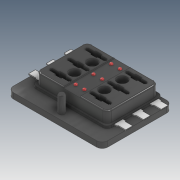
# Autodesk Inventor part: Fuse Box 6-way
Saved by Autodesk Inventor 2020 (Build 240168000, 168)
## iProperties
Created: 2021-05-27
Part Number: Fuse Box 6-way
Material: Generic
Document SubType Name: Modeling
Designer: Simon.Alvarez
Density: 1 g/cm^3
Appearance: Default
Author: Simon.Alvarez
Autodesk Inventor part; units mm, degrees
ref_plane "YZ Plane" through (0, 0, 0) normal (1, 0, 0) x (0, 1, 0)
ref_plane "XZ Plane" through (0, 0, 0) normal (0, 1, 0) x (-1, 0, 0)
ref_plane "XY Plane" through (0, 0, 0) normal (0, 0, 1) x (1, 0, 0)
sketch "Sketch1" plane through (0, 0, 0) normal (0, 1, 0) x (-1, 0, 0)
  line L0 (37.5, 31.5) -> (-37.5, 31.5)
  line L1 (-42.5, 26.5) -> (-42.5, -26.5)
  line L2 (-37.5, -31.5) -> (37.5, -31.5)
  line L3 (42.5, -26.5) -> (42.5, 26.5)
  line L4 (42.5, 31.5) -> (-42.5, -31.5) construction
  line L5 (-42.5, 31.5) -> (42.5, -31.5) construction
  arc A0 (42.5, 26.5) -> (37.5, 31.5) centre (37.5, 26.5) ccw
  arc A1 (-37.5, 31.5) -> (-42.5, 26.5) centre (-37.5, 26.5) ccw
  arc A2 (-42.5, -26.5) -> (-37.5, -31.5) centre (-37.5, -26.5) ccw
  arc A3 (37.5, -31.5) -> (42.5, -26.5) centre (37.5, -26.5) ccw
  point P0 (0, 0)
  dimension "d0" = 85
  dimension "d1" = 63
  dimension "d2" = 5
  constraints: 12 end point, 8 point on circle, 8 point on line, 8 tangent, 4 centre point, 3 equal radius, 2 midpoint, 2 parallel, 1 horizontal, 1 perpendicular
  measures "d0" distance of L4.end L5.end
  measures "d1" distance of L5.end L4.start
  measures "d2" radius of A0
extrude "Extrusion1" add sketch "Sketch1" along normal blind 5
sketch "Sketch2" plane through (0, 5, 0) normal (0, 1, 0) x (1, 0, 0)
  line L0 (37.5, 31.5) -> (-37.5, 31.5) projected
  line L1 (-30, 31.5) -> (30, 31.5)
  line L2 (34, 27.5) -> (34, -14.5)
  line L3 (30, -18.5) -> (-30, -18.5)
  line L4 (-34, -14.5) -> (-34, 27.5)
  line L5 (-42.5, 26.5) -> (-42.5, -26.5) projected
  line L6 (42.5, -26.5) -> (42.5, 26.5) projected
  line L7 (-37.5, -31.5) -> (37.5, -31.5) projected
  arc A0 (-34, -14.5) -> (-30, -18.5) centre (-30, -14.5) ccw
  arc A1 (30, -18.5) -> (34, -14.5) centre (30, -14.5) ccw
  arc A2 (34, 27.5) -> (30, 31.5) centre (30, 27.5) ccw
  arc A3 (-30, 31.5) -> (-34, 27.5) centre (-30, 27.5) ccw
  point P0 (0, 0)
  point P1 (-34, 31.5)
  point P2 (30, 31.5)
  dimension "d6" = 8.5
  dimension "d7" = 8.5
  dimension "d8" = 13
  dimension "d9" = 4
  constraints: 8 end point, 8 point on circle, 8 tangent, 4 centre point, 3 equal radius, 3 point on line, 2 parallel, 1 horizontal, 1 perpendicular
  measures "d6" distance between parallel lines of L5 L4
  measures "d7" distance between parallel lines of L6 L2
  measures "d8" distance between parallel lines of L7 L3
  measures "d9" radius of A0
extrude "Extrusion2" add sketch "Sketch2" along normal blind 2
sketch "Sketch3" plane through (0, 7, 0) normal (0, 1, 0) x (1, 0, 0)
  line L0 (-28, 29.5) -> (28, 29.5)
  line L1 (32, 25.5) -> (32, -12.5)
  line L2 (28, -16.5) -> (-28, -16.5)
  line L3 (-32, -12.5) -> (-32, 25.5)
  line L4 (30, 31.5) -> (-30, 31.5) projected
  line L5 (-34, 27.5) -> (-34, -14.5) projected
  line L6 (-30, -18.5) -> (30, -18.5) projected
  line L7 (34, -14.5) -> (34, 27.5) projected
  arc A0 (-28, 29.5) -> (-32, 25.5) centre (-28, 25.5) ccw
  arc A1 (-32, -12.5) -> (-28, -16.5) centre (-28, -12.5) ccw
  arc A2 (28, -16.5) -> (32, -12.5) centre (28, -12.5) ccw
  arc A3 (32, 25.5) -> (28, 29.5) centre (28, 25.5) ccw
  point P0 (0, 0)
  dimension "d12" = 2
  dimension "d13" = 2
  dimension "d14" = 2
  dimension "d15" = 2
  dimension "d16" = 4
  constraints: 8 end point, 8 point on circle, 8 tangent, 4 centre point, 3 equal radius, 2 parallel, 1 horizontal, 1 perpendicular
  measures "d12" distance between parallel lines of L0 L4
  measures "d13" distance between parallel lines of L5 L3
  measures "d14" distance between parallel lines of L6 L2
  measures "d15" distance between parallel lines of L7 L1
  measures "d16" radius of A0
extrude "Extrusion3" add sketch "Sketch3" along normal blind 10
fillet "Fillet1" radius 1 8 edges at (30.8284, 17, 15.3284) (32, 17, -6.5) (30.8284, 17, -28.3284) (0, 17, -29.5) (-30.8284, 17, -28.3284) (-32, 17, -6.5) (-30.8284, 17, 15.3284) (0, 17, 16.5)
sketch "Sketch4" plane through (0, 5, 0) normal (0, 1, 0) x (1, 0, 0)
  circle A0 centre (0, -25.5) radius 2.5
  line L0 (-37.5, -31.5) -> (37.5, -31.5) projected
  point P0 (0, 0)
  dimension "d20" = 5
  dimension "d21" = 6
  constraints: 1 centre point
  measures "d20" diameter of A0
  measures "d21" distance from line of L0 A0.centre
extrude "Extrusion4" add sketch "Sketch4" along normal blind 15
sketch "Sketch5" plane through (0, 17, 0) normal (0, 1, 0) x (1, 0, 0)
  line L0 (28, -16.5) -> (-28, -16.5) projected
  line L1 (-28, 29.5) -> (28, 29.5) projected
  line L2 (-7.5, -16.5) -> (7.5, -16.5)
  line L3 (7.5, -16.5) -> (7.5, 29.5)
  line L4 (7.5, 29.5) -> (-7.5, 29.5)
  line L5 (-7.5, 29.5) -> (-7.5, -16.5)
  point P0 (0, 0)
  point P1 (7.5, -16.5)
  dimension "d24" = 15
  dimension "d25" = 7.5
  constraints: 8 end point, 2 parallel, 2 point on line, 1 horizontal, 1 perpendicular
  measures "d24" distance of L3.end L4.end
  measures "d25" distance from line of point (0, 0) L3
extrude "Extrusion5" cut sketch "Sketch5" against normal blind 1
sketch "Sketch6" plane through (0, 17, 0) normal (0, 1, 0) x (1, 0, 0)
  line L0 (-13.5, -0.5) -> (13.5, -0.5)
  line L1 (13.5, -0.5) -> (13.5, 15.5)
  line L2 (13.5, 15.5) -> (-13.5, 15.5)
  line L3 (-13.5, 15.5) -> (-13.5, -0.5)
  line L4 (-13.5, -0.5) -> (13.5, 15.5) construction
  line L5 (13.5, -0.5) -> (-13.5, 15.5) construction
  line L6 (30, 31.5) -> (-30, 31.5) projected
  point P0 (0, 0)
  point P1 (0, 7.5)
  dimension "d28" = 27
  dimension "d29" = 16
  dimension "d30" = 24
  constraints: 12 end point, 4 coincident, 2 midpoint, 2 parallel, 1 horizontal, 1 perpendicular
  measures "d28" distance of L1.end L2.end
  measures "d29" distance of L2.end L0.start
  measures "d30" distance from line of point (0, 7.5) L6
hole "Hole1" at (-13.5, 17, -15.5) at (-13.5, 17, 0.5) at (13.5, 17, 0.5) at (13.5, 17, -15.5) direction (0, -1, 0) diameter 4.5 end through all counterbore diameter 9 counterbore depth 5
sketch "Sketch8" plane through (0, 16, 0) normal (0, 1, 0) x (1, 0, 0)
  circle A0 centre (-4.3463, 23.5) radius 1.5
  circle A1 centre (3.4537, 23.5) radius 1.5
  circle A2 centre (-4.3463, 7.5) radius 1.5
  circle A3 centre (3.4537, 7.5) radius 1.5
  circle A4 centre (-4.3463, -8.5) radius 1.5
  circle A5 centre (3.4537, -8.5) radius 1.5
  line L0 (7.5, 29.5) -> (-7.5, 29.5) projected
  point P0 (0, 0)
  dimension "d44" = 3
  dimension "d45" = 6
  dimension "d46" = 7.8
  dimension "d47" = 16
  dimension "d48" = 16
  dimension "d49" = 16
  dimension "d50" = 16
  dimension "d51" = 3
  dimension "d52" = 3
  dimension "d53" = 3
  dimension "d54" = 3
  dimension "d55" = 3
  constraints: 6 centre point, 4 vertical alignment, 1 horizontal alignment
  measures "d44" diameter of A0
  measures "d45" distance from line of A0.centre L0
  measures "d46" distance of A1.centre A0.centre
  measures "d47" distance of A3.centre A1.centre
  measures "d48" distance of A3.centre A5.centre
  measures "d49" distance of A2.centre A0.centre
  measures "d50" distance of A4.centre A2.centre
  measures "d51" diameter of A1
  measures "d52" diameter of A2
  measures "d53" diameter of A3
  measures "d54" diameter of A4
  measures "d55" diameter of A5
extrude "Extrusion6" add sketch "Sketch8" along normal blind 1.5
fillet "Fillet2" radius 1.5 1 edges at (-5.8463, 17.5, -23.5)
fillet "Fillet3" radius 1.5 1 edges at (1.9537, 17.5, -23.5)
fillet "Fillet4" radius 1.5 1 edges at (-5.8463, 17.5, -7.5)
fillet "Fillet5" radius 1.5 1 edges at (1.9537, 17.5, -7.5)
fillet "Fillet6" radius 1.5 1 edges at (-5.8463, 17.5, 8.5)
fillet "Fillet7" radius 1.5 1 edges at (1.9537, 17.5, 8.5)
sketch "Sketch9" plane through (0, 17, 0) normal (0, 1, 0) x (1, 0, 0)
  line L0 (-21, 26) -> (-15, 26)
  line L1 (-15, 26) -> (-15, 21)
  line L2 (-15, 21) -> (-21, 21)
  line L3 (-21, 21) -> (-21, 26)
  line L4 (-21, 26) -> (-15, 21) construction
  line L5 (-15, 26) -> (-21, 21) construction
  line L6 (-7.5, 29.5) -> (-28, 29.5) projected
  line L7 (-26.75, 22) -> (-9.25, 22)
  line L8 (-9.25, 22) -> (-9.25, 25)
  line L9 (-9.25, 25) -> (-26.75, 25)
  line L10 (-26.75, 25) -> (-26.75, 22)
  line L11 (-26.75, 22) -> (-9.25, 25) construction
  line L12 (-9.25, 22) -> (-26.75, 25) construction
  line L13 (-27.5, 22.75) -> (-8.5, 22.75)
  line L14 (-8.5, 22.75) -> (-8.5, 24.25)
  line L15 (-8.5, 24.25) -> (-27.5, 24.25)
  line L16 (-27.5, 24.25) -> (-27.5, 22.75)
  line L17 (-27.5, 22.75) -> (-8.5, 24.25) construction
  line L18 (-8.5, 22.75) -> (-27.5, 24.25) construction
  point P0 (0, 0)
  point P1 (-18, 23.5)
  point P2 (-21, 25)
  point P3 (-26.75, 24.25)
  point P4 (-26.75, 22.75)
  point P5 (-21, 22)
  point P6 (-15, 22)
  point P7 (-9.25, 22.75)
  point P8 (-9.25, 24.25)
  point P9 (-15, 25)
  dimension "d65" = 6
  dimension "d66" = 5
  dimension "d67" = 6
  dimension "d68" = 18
  dimension "d69" = 17.5
  dimension "d70" = 3
  dimension "d71" = 19
  dimension "d72" = 1.5
  constraints: 36 end point, 6 midpoint, 6 parallel, 3 horizontal, 3 perpendicular
  measures "d65" distance of L0.start L0.end
  measures "d66" distance of L0.end L1.end
  measures "d67" distance from line of point (-18, 23.5) L6
  measures "d68" horizontal distance of point (0, 0) point (-18, 23.5)
  measures "d69" distance of L8.end L9.end
  measures "d70" distance of L9.end L7.start
  measures "d71" distance of L14.end L15.end
  measures "d72" distance of L15.end L13.start
extrude "Extrusion7" cut sketch "Sketch9" against normal blind 4
pattern_linear "Rectangular Pattern1" count 3 spacing 16 along (0, 0, 1) of "Extrusion7"
mirror "Mirror1" about plane through (0, 0, 0) normal (1, 0, 0) of "Extrusion7", "Rectangular Pattern1"
chamfer "Chamfer1" distance 0.25 angle 45 1 edges at (-2.5, 20, 25.5)
thread "Thread1" size "M5x0.8" class "6g" standard "ANSI Metric M Profile" full length
sketch "Sketch10" plane through (-34, 5, -27.5) normal (-1, 0, 0) x (0, 0, 1)
  line L0 (0, 1.6341) -> (8, 1.6341)
  line L1 (8, 1.6341) -> (8, 0.8341)
  line L2 (8, 0.8341) -> (0, 0.8341)
  line L3 (0, 0.8341) -> (0, 1.6341)
  line L4 (0, 1.6341) -> (8, 0.8341) construction
  line L5 (8, 1.6341) -> (0, 0.8341) construction
  line L6 (-2, 2) -> (-2, 11) projected
  point P0 (27.5, -5)
  point P1 (4, 1.2341)
  dimension "d83" = 8
  dimension "d84" = 0.8
  dimension "d85" = 6
  constraints: 12 end point, 2 midpoint, 2 parallel, 1 horizontal, 1 perpendicular
  measures "d83" distance of L0.start L0.end
  measures "d84" distance of L0.end L1.end
  measures "d85" distance from line of L6 point (4, 1.234)
extrude "Extrusion8" add sketch "Sketch10" along normal blind 3
sketch "Sketch11" plane through (-37, 5, -27.5) normal (-1, 0, 0) x (0, 0, 1)
  line L0 (0.85, 0.8341) -> (7.15, 0.8341)
  line L1 (7.15, 0.8341) -> (7.15, 1.6341)
  line L2 (7.15, 1.6341) -> (0.85, 1.6341)
  line L3 (0.85, 1.6341) -> (0.85, 0.8341)
  line L4 (0.85, 0.8341) -> (7.15, 1.6341) construction
  line L5 (7.15, 0.8341) -> (0.85, 1.6341) construction
  line L6 (8, 1.6341) -> (0, 1.6341) projected
  line L7 (0, 1.6341) -> (0, 0.8341) projected
  point P0 (27.5, -5)
  point P1 (4, 1.2341)
  dimension "d88" = 6.3
  dimension "d89" = 0.8
  dimension "d90" = 0
  dimension "d91" = 0.85
  constraints: 12 end point, 2 midpoint, 2 parallel, 1 horizontal, 1 perpendicular
  measures "d88" distance of L1.end L2.end
  measures "d89" distance of L0.end L1.end
  measures "d90" distance between parallel lines of L2 L6
  measures "d91" distance between parallel lines of L7 L3
extrude "Extrusion9" add sketch "Sketch11" along normal blind 7
chamfer "Chamfer2" distance 0.5 angle 45 2 edges at (-44, 6.2341, -20.35) (-44, 6.2341, -26.65)
chamfer "Chamfer3" distance 0.25 angle 45 2 edges at (-44, 6.6341, -23.5) (-44, 5.8341, -23.5)
pattern_linear "Rectangular Pattern2" count 3 spacing 16 along (0, 0, 1) of "Extrusion8", "Extrusion9", "Chamfer2", "Chamfer3"
mirror "Mirror2" about plane through (0, 0, 0) normal (1, 0, 0) of "Extrusion8", "Extrusion9", "Chamfer2", "Chamfer3", "Rectangular Pattern2"
equation "\"d25\" = 0.5 * d24"
equation "\"d48\" = d47"
equation "\"d49\" = d47"
equation "\"d50\" = d49"
equation "\"d51\" = d44"
equation "\"d52\" = d44"
equation "\"d53\" = d44"
equation "\"d54\" = d44"
equation "\"d55\" = d44"
body "Solid1"
